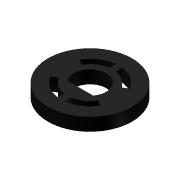
# Autodesk Inventor part: SLIPRING_SRG-1-6G_シャフト
Saved by Autodesk Inventor 2011 SP1 (Build 150282100, 282)
## iProperties
Created: 2012-05-24
Part Number: SLIPRING_SRG-1-6G_シャフト
Document SubType Name: Modeling
Designer: arihon
Density: 1 g/cm^3
Author: arihon
Autodesk Inventor part; units mm, degrees
ref_plane "YZ Plane" through (0, 0, 0) normal (1, 0, 0) x (0, 1, 0)
ref_plane "XZ Plane" through (0, 0, 0) normal (0, 1, 0) x (-1, 0, 0)
ref_plane "XY Plane" through (0, 0, 0) normal (0, 0, 1) x (1, 0, 0)
sketch "スケッチ1" plane through (0, 0, 0) normal (0, 0, 1) x (1, 0, 0)
  circle A0 centre (0, 0) radius 6.5
  arc A1 (2, -1.5) -> (-2, -1.5) centre (0, 0) ccw
  line L0 (2, -1.5) -> (-2, -1.5)
  arc A2 (-2, -1.5) -> (2, -1.5) centre (0, 0) ccw
  dimension "d0" = 13
  dimension "d1" = 5
  dimension "d2" = 4
  constraints: 4 point on circle, 3 centre point, 2 coincident, 2 end point, 1 horizontal
  measures "d0" diameter of A0
  measures "d1" diameter of A1
extrude "押し出し1" add sketch "スケッチ1" along normal blind 2 contours A0 | A2 L0
sketch "スケッチ2" plane through (0, 0, 2) normal (0, 0, 1) x (1, 0, 0)
  circle A0 centre (0, 0) radius 6.5 projected
  line L0 (0.5, -6.5) -> (0, -6.5)
  line L1 (0, -6.5) -> (-0.5, -6.5)
  arc A1 (2, -1.5) -> (-2, -1.5) centre (0, 0) ccw projected
  arc A2 (3.8971, 2.25) -> (0.5, 4.4721) centre (0, 0) ccw
  arc A3 (3.0311, 1.75) -> (0.5, 3.4641) centre (0, 0) ccw
  arc A4 (-0.5, 4.4721) -> (-3.8971, 2.25) centre (0, 0) ccw
  arc A5 (-0.5, 3.4641) -> (-3.0311, 1.75) centre (0, 0) ccw
  arc A6 (0.5, -3.4641) -> (3.0311, -1.75) centre (0, 0) ccw
  arc A7 (-3.0311, -1.75) -> (-0.5, -3.4641) centre (0, 0) ccw
  arc A8 (-3.8971, -2.25) -> (-0.5, -4.4721) centre (0, 0) ccw
  arc A9 (0.5, -4.4721) -> (3.8971, -2.25) centre (0, 0) ccw
  line L2 (-3.0311, 1.75) -> (-3.8971, 2.25)
  line L3 (-0.5, 3.4641) -> (-0.5, 4.4721)
  line L4 (0.5, 4.4721) -> (0.5, 3.4641)
  line L5 (3.0311, 1.75) -> (3.8971, 2.25)
  line L6 (-3.0311, -1.75) -> (-3.8971, -2.25)
  line L7 (3.0311, -1.75) -> (3.8971, -2.25)
  line L8 (-0.5, -4.4721) -> (-0.5, -3.4641)
  line L9 (0.5, -3.4641) -> (0.5, -4.4721)
  constraints: 20 end point, 19 point on circle, 8 centre point, 2 coincident, 2 perpendicular, 2 point on line, 1 collinear, 1 horizontal
extrude "押し出し2" cut sketch "スケッチ2" against normal through all contours L5 A3 L4 A2 | L3 A5 L2 A4 | A6 L7 A9 L9 | A7 L8 A8 L6
